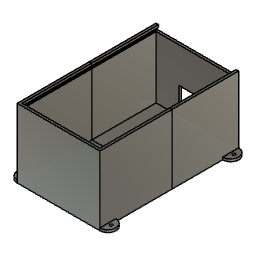
Shell (Autodesk Fusion 360 design; units mm, degrees)
Autodesk Fusion 360 part; units mm, degrees
sketch "Sketch1" plane through (0, 0, 0) normal (0, 0, 1) x (1, 0, 0)
  line L0 (0, 0) -> (103, 0)
  line L1 (103, 0) -> (103, 173)
  line L2 (103, 173) -> (0, 173)
  line L3 (0, 173) -> (0, 0)
  dimension "d1" = 103
  dimension "d2" = 173
  constraint horizontal L0
  constraint vertical L1
  constraint horizontal L2
  constraint vertical L3
  constraint coincident L0.start L3.end
  measures "d1" distance of L0.start L0.end
  measures "d2" distance of L0.start L2.end
extrude "Extrude1" add sketch "Sketch1" along normal blind 3 makes body 1
sketch "Sketch2" plane through (0, 0, 3) normal (0, 0, 1) x (-1, 0, 0)
  line L0 (0, -173) -> (0, 0)
  line L1 (0, 0) -> (-103, 0)
  line L2 (-103, 0) -> (-103, -173)
  line L3 (-103, -173) -> (0, -173)
  line L4 (0, -173) -> (-3, -173)
  line L5 (-3, -170) -> (-3, -3)
  line L6 (-3, 0) -> (0, 0)
  line L7 (0, 0) -> (0, -173)
  line L8 (0, -173) -> (-103, -173)
  line L9 (-103, -173) -> (-103, -170)
  line L10 (-100, -170) -> (-3, -170)
  line L11 (0, -170) -> (0, -173)
  line L12 (-103, -173) -> (-100, -173)
  line L13 (-100, -170) -> (-100, -3)
  line L14 (-100, 0) -> (-103, 0)
  line L15 (-103, 0) -> (-103, -173)
  line L16 (-3, -3) -> (-100, -3)
  line L17 (-103, -3) -> (-103, 0)
  line L18 (-103, 0) -> (0, 0)
  line L19 (0, 0) -> (0, -3)
  dimension "d5" = 3
  dimension "d6" = 3
  dimension "d7" = 3
  dimension "d8" = 3
  constraint horizontal L4
  constraint vertical L5
  constraint horizontal L6
  constraint vertical L7
  constraint coincident L1 L6.start
  constraint coincident L0.start L3.end
  constraint horizontal L8
  constraint vertical L9
  constraint horizontal L10
  constraint vertical L11
  constraint coincident L2 L9.end
  constraint horizontal L12
  constraint vertical L13
  constraint horizontal L14
  constraint vertical L15
  constraint coincident L1 L14.start
  constraint coincident L2.end L3.start
  constraint horizontal L16
  constraint vertical L17
  constraint horizontal L18
  constraint vertical L19
  constraint coincident L1.end L2.start
  constraint coincident L7 L19.end
  measures "d5" distance of L5 L7
  measures "d6" distance of L8 L10
  measures "d7" distance of L13 L15
  measures "d8" distance of L16 L18
extrude "Extrude2" add sketch "Sketch2" along normal blind 83 bodies 1
sketch "Sketch3" plane through (0, 173, 0) normal (0, 1, 0) x (-1, 0, 0)
  line L0 (-103, 0) -> (0, 0)
  line L1 (0, 0) -> (0, 86)
  line L2 (0, 86) -> (-103, 86)
  line L3 (-103, 86) -> (-103, 0)
  line L4 (-71.5, 3) -> (-31.5, 3)
  line L5 (-31.5, 3) -> (-31.5, 36)
  line L6 (-31.5, 36) -> (-71.5, 36)
  line L7 (-71.5, 36) -> (-71.5, 3)
  dimension "d11" = 3
  dimension "d12" = 33
  dimension "d13" = 40
  dimension "d14" = 31.5
  constraint horizontal L4
  constraint vertical L5
  constraint horizontal L6
  constraint vertical L7
  measures "d11" distance of L0 L4
  measures "d12" distance of L4.start L6.end
  measures "d13" distance of L5.end L6.end
  measures "d14" distance of L1 L5
extrude "Extrude3" cut sketch "Sketch3" against normal blind 3 contours L4 L5 L6 L7 bodies 1
sketch "Sketch4" plane through (0, 173, 0) normal (0, 1, 0) x (-1, 0, 0)
  line L0 (-31.5, 3) -> (-71.5, 3)
  line L1 (-71.5, 3) -> (-71.5, 36)
  line L2 (-71.5, 36) -> (-31.5, 36)
  line L3 (-31.5, 36) -> (-31.5, 3)
  line L4 (-103, 0) -> (0, 0)
  line L5 (0, 0) -> (0, 86)
  line L6 (0, 86) -> (-103, 86)
  line L7 (-103, 86) -> (-103, 0)
  line L8 (-100, 86) -> (-3, 86)
  line L9 (-3, 86) -> (-3, 80)
  line L10 (-3, 80) -> (-100, 80)
  line L11 (-100, 80) -> (-100, 86)
  dimension "d17" = 6
  dimension "d18" = 3
  dimension "d19" = 3
  constraint horizontal L8
  constraint vertical L9
  constraint horizontal L10
  constraint vertical L11
  constraint coincident L6 L8.start
  measures "d17" distance of L8.start L10.end
  measures "d18" distance of L7 L11
  measures "d19" distance of L5 L9
extrude "Extrude4" cut sketch "Sketch4" against normal blind 3 contours L6 L8 L9 L10 L11 bodies 1
sketch "Sketch5" plane through (0, 173, 0) normal (0, 1, 0) x (-1, 0, 0)
  line L0 (-100, 80) -> (-100, 86)
  line L1 (-100, 86) -> (-103, 86)
  line L2 (-103, 86) -> (-103, 0)
  line L3 (-103, 0) -> (0, 0)
  line L4 (0, 0) -> (0, 86)
  line L5 (0, 86) -> (-3, 86)
  line L6 (-3, 86) -> (-3, 80)
  line L7 (-3, 80) -> (-100, 80)
  line L8 (-31.5, 3) -> (-71.5, 3)
  line L9 (-71.5, 3) -> (-71.5, 36)
  line L10 (-71.5, 36) -> (-31.5, 36)
  line L11 (-31.5, 36) -> (-31.5, 3)
  line L12 (-101.5, 83) -> (-1.5, 83)
  line L13 (-1.5, 83) -> (-1.5, 80)
  line L14 (-1.5, 80) -> (-101.5, 80)
  line L15 (-101.5, 80) -> (-101.5, 83)
  dimension "d22" = 1.5
  dimension "d23" = 1.5
  dimension "d24" = 3
  dimension "d25" = 3
  constraint horizontal L12
  constraint vertical L13
  constraint horizontal L14
  constraint vertical L15
  measures "d22" distance of L2 L15
  measures "d23" distance of L4 L13
  measures "d24" distance of L12 L14
  measures "d25" distance of L1 L12
extrude "Extrude5" cut sketch "Sketch5" against normal blind 171.5 contours L0 L12 L14 L15 | L0 L6 L7 L12 L14 | L6 L12 L13 L14 bodies 1
sketch "Sketch6" plane through (0, 0, 0) normal (0, 0, -1) x (1, 0, 0)
  line L0 (0, 0) -> (0, -173)
  line L1 (0, -173) -> (103, -173)
  line L2 (103, -173) -> (103, 0)
  line L3 (103, 0) -> (0, 0)
  circle A0 centre (0, -10) radius 10
  circle A1 centre (0, -163) radius 10
  circle A2 centre (103, -163) radius 10
  circle A3 centre (103, -10) radius 10
  circle A4 centre (-4, -10) radius 1.75
  circle A5 centre (-4, -163) radius 1.75
  circle A6 centre (107, -163) radius 1.75
  circle A7 centre (107, -10) radius 1.75
  dimension "d28" = 20
  dimension "d29" = 20
  dimension "d30" = 20
  dimension "d31" = 20
  dimension "d32" = 3.5
  dimension "d33" = 4
  dimension "d34" = 3.5
  dimension "d35" = 4
  dimension "d36" = 3.5
  dimension "d37" = 4
  dimension "d38" = 3.5
  dimension "d39" = 4
  constraint coincident L0 A0.centre
  constraint coincident L0.start A0
  constraint coincident L0 A1.centre
  constraint coincident L0.end A1
  constraint coincident L2 A2.centre
  constraint coincident L1.end A2
  constraint coincident L2 A3.centre
  constraint coincident L2.end A3
  measures "d28" diameter of A0
  measures "d29" diameter of A1
  measures "d30" diameter of A2
  measures "d31" diameter of A3
  measures "d32" diameter of A4
  measures "d33" distance of A0.centre A4.centre
  measures "d34" diameter of A5
  measures "d35" distance of L0 A5.centre
  measures "d36" diameter of A6
  measures "d37" distance of L2 A6.centre
  measures "d38" diameter of A7
  measures "d39" distance of L2 A7.centre
extrude "Extrude6" add sketch "Sketch6" against normal blind 3 contours L0 A0 | L2 A3 | L0 A1 | L2 A2 picked at (-0.75, -10) picked at (103.75, -10) picked at (-0.75, -163) picked at (103.75, -163) bodies 1
sketch "Sketch7" plane through (0, 0, 0) normal (0, 0, -1) x (1, 0, 0)
  circle A0 centre (107, -10) radius 1.75
  circle A1 centre (107, -163) radius 1.75
  circle A2 centre (-4, -10) radius 1.75
  circle A3 centre (-4, -163) radius 1.75
  line L0 (0, -173) -> (103, -173)
  arc A4 (103, -173) -> (103, -153) centre (103, -163) ccw
  line L1 (103, -153) -> (103, -20)
  arc A5 (103, -20) -> (103, 0) centre (103, -10) ccw
  line L2 (103, 0) -> (0, 0)
  arc A6 (0, 0) -> (0, -20) centre (0, -10) ccw
  line L3 (0, -20) -> (0, -153)
  arc A7 (0, -153) -> (0, -173) centre (0, -163) ccw
ref_plane "WorkPlane2" through (0, 90, 0) normal (0, 1, 0) x (0, 0, 1)
split "Split1" by plane through (0, 90, 0) normal (0, 1, 0) bodies 1 makes body 2 at (34.3333, 132, 0)
